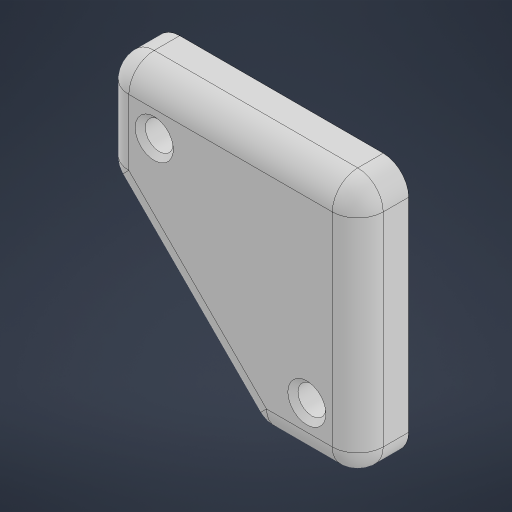
# Autodesk Inventor part: 모서리 결합
Saved by Autodesk Inventor 2024 (Build 280153000, 153)
## iProperties
Created: 2024-01-11
Part Number: 모서리 결합
Material: 일반
Document SubType Name: Modeling
Designer: KBU
Density: 1 g/cm^3
Appearance: 기본값
Author: KBU
Autodesk Inventor part; units mm, degrees
ref_plane "YZ Plane" through (0, 0, 0) normal (1, 0, 0) x (0, 1, 0)
ref_plane "XZ Plane" through (0, 0, 0) normal (0, 1, 0) x (-1, 0, 0)
ref_plane "XY Plane" through (0, 0, 0) normal (0, 0, 1) x (1, 0, 0)
sketch "스케치1" plane through (0, 0, 0) normal (0, 0, 1) x (1, 0, 0)
  line L0 (5, -25) -> (25, -25)
  line L1 (25, -25) -> (25, 25)
  line L2 (25, 25) -> (-25, 25)
  line L3 (-25, 25) -> (-25, 5)
  line L4 (-10, -10) -> (25, 25) construction
  line L5 (25, -25) -> (-25, 25) construction
  line L6 (5, -25) -> (-25, 5)
  point P0 (0, 0)
  dimension "d0" = 50
  dimension "d1" = 50
  dimension "d2" = 20
  dimension "d3" = 20
  constraints: 14 end point, 2 midpoint, 2 parallel, 1 horizontal, 1 perpendicular, 1 point on line
  measures "d0" distance of L0.end L1.end
  measures "d1" distance of L1.end L2.end
  measures "d2" distance from line of L3.end L2
  measures "d3" distance from line of L0.start L1
extrude "돌출1" add sketch "스케치1" along normal blind 10
fillet "모깎기1" radius 5 5 edges at (25, 25, 5) (25, -25, 5) (-25, 25, 5) (-25, 5, 5) (5, -25, 5)
fillet "모깎기2" radius 5 10 edges at (23.5355, 23.5355, 10) (0, 25, 10) (-23.5355, 23.5355, 10) (-25, 13.5355, 10) (-24.6194, 5.1577, 10) (-10, -10, 10) (5.1577, -24.6194, 10) (13.5355, -25, 10) (23.5355, -23.5355, 10) (25, 0, 10)
sketch "스케치2" plane through (0, 0, 0) normal (0, 0, -1) x (-1, 0, 0)
  line L0 (25, 20) -> (25, 7.0711) projected
  line L1 (-20, 25) -> (20, 25) projected
  line L2 (-25, -20) -> (-25, 20) projected
  line L3 (-7.0711, -25) -> (-20, -25) projected
  line L4 (-15, 15) -> (15, 15) construction
  line L5 (-15, -15) -> (-15, 15) construction
  circle A0 centre (-15, -15) radius 2.75
  circle A1 centre (15, 15) radius 2.75
  point P0 (0, 0)
  point P1 (-25, 0)
  dimension "d8" = 10
  dimension "d10" = 10
  dimension "d11" = 10
  dimension "d12" = 10
  dimension "d13" = 5.5
  dimension "d14" = 5.5
  constraints: 4 end point, 2 centre point, 2 coincident, 1 horizontal, 1 midpoint
  measures "d8" distance between parallel lines of L1 L4
  measures "d10" distance between parallel lines of L2 L5
  measures "d11" distance from line of L0 L4.end
  measures "d12" distance from line of L3 L5.start
  measures "d13" diameter of A0
  measures "d14" diameter of A1
extrude "돌출2" cut sketch "스케치2" against normal blind 10
chamfer "모따기1" distance 1 angle 45 2 edges at (-12.25, 15, 10) (17.75, -15, 10)
equation "\"d13\" = d14"
